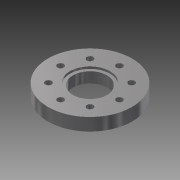
# Autodesk Inventor part: 03
Saved by Autodesk Inventor 2013 (Build 170138000, 138)
## iProperties
Created: 2014-02-07
Material: アルミニウム 6061
Document SubType Name: Modeling
Designer: andou
Density: 2.71 g/cm^3
Mass: 1.57929 g
Surface Area: 8.26239 cm^2
Volume: 0.582765 cm^3
Part Number: 03
Author: andou
Title: Bearing-Holder
Autodesk Inventor part; units mm, degrees
ref_plane "YZ Plane" through (0, 0, 0) normal (1, 0, 0) x (0, 1, 0)
ref_plane "XZ Plane" through (0, 0, 0) normal (0, 1, 0) x (-1, 0, 0)
ref_plane "XY Plane" through (0, 0, 0) normal (0, 0, 1) x (1, 0, 0)
sketch "スケッチ1" plane through (0, 0, 0) normal (0, 0, 1) x (1, 0, 0)
  circle A0 centre (0, 0) radius 10
  dimension "d0" = 20
  constraints: 1 centre point, 1 coincident
  measures "d0" diameter of A0
extrude "押し出し1" add sketch "スケッチ1" along normal blind 3
sketch "スケッチ5" plane through (0, 0, 3) normal (0, 0, 1) x (1, 0, 0)
  circle A0 centre (0, 7) radius 1
  circle A1 centre (0, 0) radius 10 projected
  dimension "d30" = 2
  dimension "d77" = 0
  dimension "d78" = 7
  constraints: 1 centre point
  measures "d30" diameter of A0
  measures "d77" horizontal distance of A0.centre A1.centre
  measures "d78" distance of A1.centre A0.centre
hole "穴4" at (0, 7, 3) direction (0, 0, -1) diameter 1.5 end through all
sketch "スケッチ6" plane through (0, 0, 0) normal (0, 0, -1) x (-1, 0, 0)
  circle A0 centre (0, 0) radius 10 projected
  circle A1 centre (0, 0) radius 4.05
  dimension "d66" = 8.1
  constraints: 1 centre point, 1 coincident
  measures "d66" diameter of A1
hole "穴5" at (0, 0, 0) direction (0, 0, 1) diameter 8.1 end through all
sketch "スケッチ2" plane through (0, 0, 3) normal (0, 0, 1) x (1, 0, 0)
  circle A0 centre (0, 0) radius 10 projected
  circle A1 centre (0, 0) radius 4.75
  dimension "d3" = 9.5
  constraints: 1 centre point, 1 coincident
  measures "d3" diameter of A1
extrude "押し出し4" cut sketch "スケッチ2" against normal blind 0.5 contours A1
pattern_circular "円形状パターン3" count 8 over 360 about axis through (0, 0, 28.4429) along (0, 0, -1) of "穴4"
